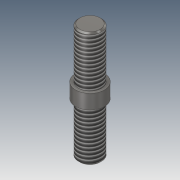
# Autodesk Inventor part: 200-60-DIFFERENTIAL-BAR-04
Saved by Autodesk Inventor 2018.2 (Build 222227000, 227)
## iProperties
Manager: feesmrt
Company: FRANCOR
Part Number: 200-60-DIFFERENTIAL-BAR-04
Project: Rescue Robot
Cost Center: -
Material: Edelstahl
Document SubType Name: Modeling
Designer: feesmrt
Engineer: feesmrt
Authority: feesmrt
Density: 8 g/cm^3
Appearance: Halbpoliert
Description: Differential Befestigungsbolzen
Stock Number: 200-60-DIFFERENTIAL-BAR-04
Subject: Rescue Robot
Author: feesmrt
Revision Number: 1
Title: Differential Befestigungsbolzen
Autodesk Inventor part; units mm, degrees
ref_plane "YZ Plane" through (0, 0, 0) normal (1, 0, 0) x (0, 1, 0)
ref_plane "XZ Plane" through (0, 0, 0) normal (0, 1, 0) x (-1, 0, 0)
ref_plane "XY Plane" through (0, 0, 0) normal (0, 0, 1) x (1, 0, 0)
sketch "Skizze1" plane through (0, 0, 0) normal (1, 0, 0) x (0, 1, 0)
  line L0 (0, 25.5) -> (0, -30.5) projected
  line L1 (-1, 0) -> (6, 0) construction
  line L2 (0, 17.5) -> (4, 17.5)
  line L3 (4, 17.5) -> (4, 0)
  line L4 (4, 0) -> (5, 0)
  line L5 (5, 0) -> (5, -5)
  line L6 (5, -5) -> (4, -5)
  line L7 (4, -5) -> (4, -22.5)
  line L8 (4, -22.5) -> (0, -22.5)
  line L9 (0, -22.5) -> (0, 17.5)
  point P0 (0, 0)
  dimension "d1" = 5
  dimension "d2" = 40
  dimension "d3" = 8
  dimension "d4" = 10
  constraints: 16 end point, 6 point on line, 4 perpendicular, 1 collinear, 1 horizontal, 1 vertical
  measures "d1" distance between parallel lines of L1 L6
  measures "d2" distance between parallel lines of L2 L8
  measures "d3" diameter of L3 L0
  measures "d4" diameter of L5 L0
revolve "Grundkörper" add sketch "Skizze1" angle 360 about axis through (0, 0, 0) along (0, 0, -1)
chamfer "Gewindefase" distance 0.5 angle 45 2 edges at (0, -4, 17.5) (0, -4, -22.5)
thread "M8-1" size "M8x1.25" class "6g" standard "ANSI Metric M Profile" full length
thread "M8-2" size "M8x1.25" class "6g" standard "ANSI Metric M Profile" full length
